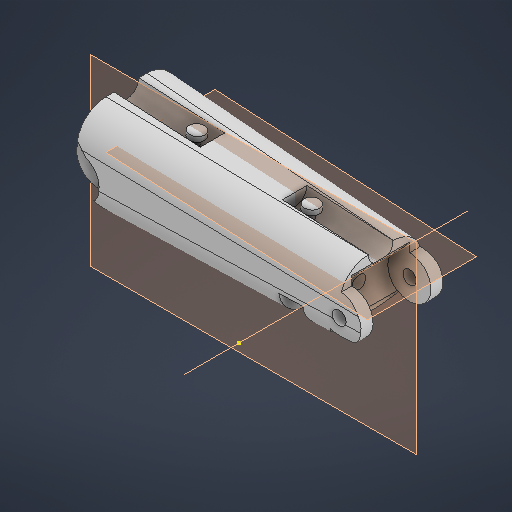
# Autodesk Inventor part: falange1_corazon_V13
Saved by Autodesk Inventor 2026.1 (Build 301233020, 233B)
## iProperties
Created: 2026-01-14
Part Number: falange1_corazon_V13
Material: Generic
Document SubType Name: Modeling
Designer: user
Density: 1 g/cm^3
Appearance: Default
Author: user
Autodesk Inventor part; units mm, degrees
ref_plane "YZ Plane" through (0, 0, 0) normal (1, 0, 0) x (0, 1, 0)
sketch "Sketch1" plane through (0, 0, 0) normal (0, 0, 1) x (1, 0, 0)
  circle A0 centre (59, 0) radius 1.575
  arc A1 (0, 5) -> (2.867882, -4.09576) centre (0, 0) ccw
  line L0 (0, 5) -> (0, 12.477091)
  arc A2 (56.175136, -4.034324) -> (59, 4.925) centre (59, 0) ccw
  line L1 (59, 4.925) -> (59, 9.275)
  line L2 (2.867882, -4.09576) -> (5.267598, -7.522909)
  line L3 (5.267598, -7.522909) -> (53.732402, -7.522909)
  line L4 (56.175136, -4.034324) -> (53.732402, -7.522909)
  line L5 (0, 12.477091) -> (59, 9.275)
  dimension "d39" = 3.15
  dimension "d46" = 10
  dimension "d57" = 12.47709
  dimension "d131" = 59
  dimension "d132" = 9.85
  dimension "d133" = 4.35
  dimension "d188" = 4.18378
  dimension "d189" = 0
  dimension "d191" = 55
  dimension "d192" = 0
  dimension "d193" = 7.47709
  dimension "d194" = 4.25878
  dimension "d195" = 55
  constraints: 12 end point, 4 point on circle, 3 centre point, 2 coincident, 2 vertical, 1 horizontal
  measures "d39" diameter of A0
  measures "d46" diameter of A1
  measures "d57" distance of L0.end point (0, 0)
  measures "d131" distance of A0.centre point (0, 0)
  measures "d132" diameter of A2
  measures "d133" distance of L1.start L1.end
  measures "d188" distance of L2.start L2.end
  measures "d189" vertical distance of point (0, 0) A0.centre
  measures "d191" angle of L3 L2
  measures "d192" distance from line of A0.centre L1
  measures "d193" distance of L0.start L0.end
  measures "d194" distance of L4.start L3.end
  measures "d195" angle of L3 L4
extrude "Extrusion1" add sketch "Sketch1" along normal mid plane 23
sketch "Sketch3" plane through (0, 0, 11.5) normal (0, 0, 1) x (1, 0, 0)
  circle A0 centre (0, 0) radius 1.575
  circle A1 centre (0, 0) radius 5
  dimension "d49" = 3.15
  dimension "d50" = 10
  constraints: 2 centre point, 2 coincident
  measures "d49" diameter of A0
  measures "d50" diameter of A1
sketch "Sketch4" plane through (0, 0, -11.5) normal (0, 0, -1) x (-1, 0, 0)
  circle A0 centre (0, 0) radius 1.5
  circle A1 centre (0, 0) radius 5
  dimension "d51" = 10
  dimension "d52" = 3
  constraints: 2 centre point, 2 coincident
  measures "d51" diameter of A1
  measures "d52" diameter of A0
extrude "Extrusion3" cut sketch "Sketch3" against normal blind 4.945 contours A0 | A1
extrude "Extrusion4" cut sketch "Sketch4" against normal blind 4.945 contours A0 | A1
sketch "Sketch8" plane through (0, 0, 11.5) normal (0, 0, 1) x (1, 0, 0)
  line L0 (50.732402, -7.522909) -> (45.361452, -7.522909)
  line L1 (45.361452, -7.522909) -> (45.361452, -1.697299)
  line L2 (45.361452, -1.697299) -> (50.732402, -1.697299)
  line L3 (50.732402, -1.697299) -> (50.732402, -7.522909)
  point P0 (0, 0)
  point P1 (53.732402, -7.522909)
  dimension "d67" = 5.82561
  dimension "d90" = 5.37095
  dimension "d197" = 3
  constraints: 8 end point, 2 parallel, 1 horizontal, 1 perpendicular
  measures "d67" distance of L2.end L0.start
  measures "d90" distance of L1.end L2.end
  measures "d197" distance of point (53.732, -7.523) L0.start
extrude "Extrusion5" cut sketch "Sketch8" against normal through all
sketch "Sketch11" plane through (45.361452, -7.522909, 11.5) normal (1, 0, 0) x (0, 0, -1)
  circle A0 centre (11.5, 2.912805) radius 1.5
  point P0 (11.5, 7.522909)
  point P1 (11.5, 0)
  dimension "d75" = 2.91281
  dimension "d76" = 3
  constraints: 1 centre point
  measures "d75" distance of point (11.5, 0) A0.centre
  measures "d76" diameter of A0
extrude "Extrusion8" cut sketch "Sketch11" against normal through all
sketch "Sketch14" plane through (0, 12.477091, -11.5) normal (-1, 0, 0) x (0, 0, 1)
  circle A0 centre (11.5, -12.477091) radius 1.5
  line L0 (0, 0) -> (23, 0)
  dimension "d92" = 3
  dimension "d166" = 12.47709
  constraints: 1 centre point, 1 coincident
  measures "d92" diameter of A0
  measures "d166" distance from line of L0 point (11.5, -12.477)
sketch "Sketch15" plane through (0, 0, 0) normal (0, 0, 1) x (1, 0, 0)
  circle A0 centre (0, 0) radius 5
  dimension "d93" = 10
  constraints: 1 centre point, 1 coincident
  measures "d93" diameter of A0
extrude "Extrusion11" cut sketch "Sketch15" along normal mid plane 3.825
extrude "Extrusion12" cut sketch "Sketch3" against normal through all contours A0
sketch "Sketch16" plane through (0, 0, -1.9125) normal (0, 0, 1) x (1, 0, 0)
  point P0 (0, 0)
sketch "Sketch17" plane through (0, 0, 0) normal (0, 0, 1) x (1, 0, 0)
  circle A0 centre (0, 0) radius 1.575
  line L0 (-1.651749, 2.630563) -> (1.45226, 2.745738)
  line L1 (1.45226, 2.745738) -> (3.104008, 0.115175)
  line L2 (3.104008, 0.115175) -> (1.651749, -2.630563)
  line L3 (1.651749, -2.630563) -> (-1.45226, -2.745738)
  line L4 (-1.45226, -2.745738) -> (-3.104008, -0.115175)
  line L5 (-3.104008, -0.115175) -> (-1.651749, 2.630563)
  dimension "d102" = 5.38
  constraints: 12 end point, 1 coincident, 13 other
  measures "d102" distance between parallel lines of L3 L0
extrude "Extrusion13" cut sketch "Sketch17" along normal mid plane 8.085 contours A0 | L0 L1 L2 L3 L4 L5
extrude "Extrusion14" cut sketch "Sketch14" against normal through all
sketch "Sketch18" plane through (0, 0, 0) normal (0, 0, 1) x (1, 0, 0)
  circle A0 centre (59, 0) radius 5.075
  arc A1 (56.175136, -4.034324) -> (59, 4.925) centre (59, 0) ccw
  point P0 (0, 0)
  dimension "d103" = 10.15
  dimension "d198" = 0
  constraints: 1 centre point
  measures "d103" diameter of A0
  measures "d198" distance of A1.centre A0.centre
extrude "Extrusion15" cut sketch "Sketch18" along normal mid plane 13.41
ref_plane "Work Plane1" through (0, 12.477091, -11.5) normal (0, 1, 0) x (-1, 0, 0)
sketch "Sketch26" plane through (0, 12.477091, -11.5) normal (-1, 0, 0) x (0, 0, 1)
  line L0 (0, 0) -> (23, 0)
  circle A0 centre (11.5, 0) radius 2.860389
  point P0 (11.5, -12.477091)
  dimension "d146" = 5.72078
  constraints: 1 centre point, 1 midpoint
  measures "d146" diameter of A0
sketch "Sketch28" plane through (59, 4.925, -11.5) normal (1, 0, 0) x (0, 0, -1)
  line L0 (0, 4.35) -> (-23, 4.35)
  circle A0 centre (-11.5, 4.35) radius 2.860389
  point P0 (-11.5, -4.925)
  dimension "d147" = 5.72078
  constraints: 1 centre point, 1 midpoint
  measures "d147" diameter of A0
sketch "Sketch29" plane through (0, 12.477091, 11.5) normal (0.054193, 0.9985305, 0) x (0.9985305, -0.054193, 0)
  line L0 (0, 23) -> (0, 0) projected
  line L1 (0, 11.5) -> (20, 11.5)
  point P0 (0.676171, 11.5)
  dimension "d144" = 20
  constraints: 2 end point, 1 horizontal, 1 midpoint
  measures "d144" distance of L1.start L1.end
sketch "Sketch30" plane through (0, 12.477091, 11.5) normal (0.054193, 0.9985305, 0) x (0.9985305, -0.054193, 0)
  line L0 (59.086829, 23) -> (59.086829, 0)
  line L1 (59.086829, 11.5) -> (39.086829, 11.5)
  point P0 (0.676171, 11.5)
  dimension "d145" = 20
  constraints: 2 end point, 1 horizontal, 1 midpoint
  measures "d145" distance of L1.start L1.end
sweep "Sweep2" cut profiles "Sketch26" path "Sketch29" path curves L1
sweep "Sweep3" cut profiles "Sketch28" path "Sketch30" path curves L1
ref_plane "Work Plane3" through (58.845215, 6.423012, 0) normal (0.054193, 0.9985305, 0) x (0.9985305, -0.054193, 0)
sketch "Sketch31" plane through (58.845215, 6.423012, 0) normal (0.054193, 0.9985305, 0) x (0.9985305, -0.054193, 0)
  line L0 (0.22761, -6.705) -> (0.22761, 6.705)
  line L1 (0.22761, 0) -> (-16.01239, 0)
  circle A0 centre (-16.01239, 0) radius 0.732091
  point P0 (-58.410659, 0)
  dimension "d152" = 16.24
  dimension "d153" = 1.46418
  constraints: 2 end point, 1 centre point, 1 coincident, 1 midpoint
  measures "d152" distance of L1.start L1.end
  measures "d153" diameter of A0
extrude "Extrusion23" add sketch "Sketch31" along normal mid plane 3.3575
sketch "Sketch32" plane through (58.845215, 6.423012, 0) normal (0.054193, 0.9985305, 0) x (0.9985305, -0.054193, 0)
  ellipse E0 centre (-59.086829, 0) end of major axis (-59.086829, -2.860389) minor radius 0.155013 (-59.086829, -2.860389) -> (-59.086829, 2.860389) ccw
  line L0 (-58.931816, 0) -> (-42.691816, 0)
  circle A0 centre (-42.691816, 0) radius 0.732091
  point P0 (-58.410659, 0)
  point P1 (-43.9139, -2.860389)
  point P2 (-43.9139, 2.860389)
  dimension "d156" = 16.24
  dimension "d157" = 1.46418
  constraints: 2 end point, 1 centre point, 1 coincident, 1 horizontal, 2 other
  measures "d156" distance of L0.start L0.end
  measures "d157" diameter of A0
extrude "Extrusion24" add sketch "Sketch32" along normal mid plane 3.3575
sketch "Sketch33" plane through (16.307111, 10.412892, 0) normal (0.054193, 0.9985305, 0) x (0.9985305, -0.054193, 0)
  circle A0 centre (0, 0) radius 0.732091
  circle A1 centre (0, 0) radius 1.774025
  point P0 (-15.718842, 0)
  dimension "d160" = 3.54805
  constraints: 1 centre point, 1 coincident
  measures "d160" diameter of A1
extrude "Extrusion25" add sketch "Sketch33" along normal up to surface (1.177435 mm away) contours A0 | A1
sketch "Sketch34" plane through (42.947332, 8.967054, 0) normal (0.054193, 0.9985305, 0) x (0.9985305, -0.054193, 0)
  circle A0 centre (0, 0) radius 0.732091
  circle A1 centre (0, 0) radius 1.774025
  point P0 (-42.398269, 0)
  dimension "d163" = 3.54805
  constraints: 1 centre point, 1 coincident
  measures "d163" diameter of A1
extrude "Extrusion26" add sketch "Sketch34" along normal up to surface (1.177435 mm away) contours A0 | A1
chamfer "Chamfer1" distance 2 angle 45 1 edges at (59, 5.075, 0)
chamfer "Chamfer2" distance 2 angle 45 2 edges at (0, 5, -9.0275) (0, 5, 9.0275)
sketch "Sketch35" plane through (50.732402, -7.522909, 11.5) normal (-1, 0, 0) x (0, 0, 1)
  line L0 (0, 5.82561) -> (-23, 5.82561)
  line L1 (0, 5.82561) -> (0, 0)
  line L2 (-23, 5.82561) -> (0, 5.82561)
  circle A0 centre (-11.5, 1.996968) radius 1
  point P0 (-11.5, 7.522909)
  dimension "d173" = 2
  constraints: 2 end point, 1 centre point, 1 perpendicular
  measures "d173" diameter of A0
ref_plane "Work Plane4" through (50.732402, -1.697299, 11.5) normal (-0.7071068, 0.7071068, 0) x (0, 0, -1)
sketch "Sketch36" plane through (50.732402, -1.697299, 11.5) normal (-0.7071068, 0.7071068, 0) x (0, 0, -1)
  point P0 (11.5, 34.673054)
sketch3d "3D Sketch1"
sketch "Sketch38" plane through (5.267598, -7.522909, -11.5) normal (0, -1, 0) x (1, 0, 0)
  line L0 (-5.267598, 23) -> (-5.267598, 18.055)
  line L1 (-5.267598, 23) -> (58.657402, 21)
  line L2 (58.657402, 21) -> (58.657402, 11.5)
  line L3 (58.657402, 18.205) -> (58.657402, 23)
  line L4 (-43.701645, 11.5) -> (75.717244, 11.5)
  line L5 (-3.615849, 13.4125) -> (-3.615849, 15.5425)
  line L6 (-5.267598, 0) -> (58.657402, 2)
  line L7 (58.657402, 2) -> (58.657402, 11.5)
  line L8 (-5.267598, 23) -> (-26.641804, 23)
  line L9 (-26.641804, 23) -> (-26.641804, 11.5)
  line L10 (-5.267598, 0) -> (-26.641804, 0)
  line L11 (-26.641804, 0) -> (-26.641804, 11.5)
  point P0 (-5.267598, 11.5)
  dimension "d179" = 9.5
  dimension "d196" = 0
  constraints: 16 end point, 3 symmetric about line, 2 perpendicular, 2 point on line, 1 collinear, 1 horizontal
  measures "d179" distance of L1.end L2.end
  measures "d196" distance between parallel lines of L3 L2
extrude "Extrusion27" cut sketch "Sketch38" against normal through all keep common part
fillet "Fillet1" radius 6.7625 2 edges at (29.5, 10.876, 10.577) (29.5, 10.876, -10.577)
fillet "Fillet2" radius 6.7625 4 edges at (25.3145, -7.5229, 10.708) (25.3145, -7.5229, -10.708) (52.2324, -7.5229, 9.8658) (52.2324, -7.5229, -9.8658)
extrude "Extrusion28" cut sketch "Sketch35" against normal blind 10
equation "\"d46\" = diametroFueraUnion"
equation "\"d132\" = diametroFueraUnion - tolerancia"
equation "\"d49\" = diametroDentroUnion + tolerancia"
equation "\"d50\" = diametroFueraUnion"
equation "\"d51\" = diametroFueraUnion"
equation "\"d52\" = diametroDentroUnion"
equation "\"d93\" = diametroFueraUnion"
equation "\"d103\" = diametroFueraUnion + tolerancia"
equation "\"diametroDentroUnion\" = 3"
equation "\"diametroFueraUnion\" = 10"
equation "\"tolerancia\" = 0.15"
body "Solid1"
